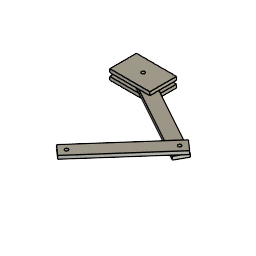
2-Link Manipulator (Autodesk Fusion 360 design; units mm, degrees)
part number: 2025-09-27-21-11-09-060
part number: 2025-09-28-14-52-39-258
part number: 2025-09-28-14-52-39-267
part number: 2025-09-28-14-52-39-272
Autodesk Fusion 360 part; units mm, degrees
sketch "草图1" plane through (0, 0, 0) normal (0, 0, 1) x (1, 0, 0)
  line L0 (30, 20) -> (-30, 20)
  line L1 (-30, 20) -> (-30, -20)
  line L2 (-30, -20) -> (30, -20)
  line L3 (30, -20) -> (30, 20)
  line L4 (30, 20) -> (-30, -20) construction
  line L5 (-30, 20) -> (30, -20) construction
  circle A0 centre (0, 0) radius 2.5
  dimension "d1" = 5
  constraint horizontal L0
  constraint perpendicular L0 L1
  constraint parallel L0 L2
  constraint parallel L1 L3
  constraint coincident L4 A0.centre
  constraint coincident L5 A0.centre
  constraint coincident A0.centre origin
  measures "d1" diameter of A0
sketch "草图3" plane through (0, 0, 0) normal (0, 0, 1) x (1, 0, 0)
  line L0 (59.3105, 8.9123) -> (219.3105, 8.9123)
  line L1 (219.3105, 8.9123) -> (219.3105, -11.0877)
  line L2 (219.3105, -11.0877) -> (59.3105, -11.0877)
  line L3 (59.3105, -11.0877) -> (59.3105, 8.9123)
  circle A0 centre (70, 0) radius 2.5
  circle A1 centre (209.3105, 0) radius 2.5
  dimension "d6" = 160
  dimension "d7" = 20
  dimension "d8" = 5
  dimension "d10" = 5
  constraint horizontal L0
  constraint vertical L1
  constraint horizontal L2
  constraint vertical L3
  measures "d6" distance of L0.start L0.end
  measures "d7" distance of L0.start L2.end
  measures "d8" diameter of A0
  measures "d10" diameter of A1
extrude "拉伸3" add sketch "草图3" along normal blind 5 makes body 1
sketch "草图4" plane through (0, 0, 0) normal (0, 0, 1) x (1, 0, 0)
  line L0 (-33, -75) -> (107, -75)
  line L1 (107, -75) -> (107, -95)
  line L2 (107, -95) -> (-33, -95)
  line L3 (-33, -95) -> (-33, -75)
  circle A0 centre (-23, -85) radius 2.5
  circle A1 centre (97, -85) radius 2.5
  dimension "d13" = 140
  dimension "d14" = 20
  dimension "d15" = 5
  dimension "d16" = 5
  constraint horizontal L0
  constraint vertical L1
  constraint horizontal L2
  constraint vertical L3
  measures "d13" distance of L0.start L0.end
  measures "d14" distance of L0.start L2.end
  measures "d15" diameter of A0
  measures "d16" diameter of A1
extrude "拉伸4" add sketch "草图4" along normal blind 5 separate body makes body 2
sketch "草图5" plane through (0, 0, 0) normal (0, 0, 1) x (1, 0, 0)
  line L0 (-30, 20) -> (30, 20)
  line L1 (30, 20) -> (30, -20)
  line L2 (30, -20) -> (-30, -20)
  line L3 (-30, -20) -> (-30, 20)
  line L4 (-30, 20) -> (30, -20) construction
  line L5 (30, 20) -> (-30, -20) construction
  circle A0 centre (0, 0) radius 2.5
  dimension "d19" = 60
  dimension "d20" = 40
  dimension "d21" = 5
  constraint horizontal L0
  constraint perpendicular L0 L1
  constraint parallel L0 L2
  constraint parallel L1 L3
  constraint coincident L4 A0.centre
  constraint coincident L5 A0.centre
  constraint coincident A0.centre origin
  measures "d19" distance of L1.end L2.end
  measures "d20" distance of L0.end L1.end
  measures "d21" diameter of A0
extrude "拉伸5" add sketch "草图5" along normal blind 5 separate body makes body 3
sketch "草图6" plane through (0, 0, 0) normal (0, 0, 1) x (1, 0, 0)
  circle A0 centre (76.9556, 57.3858) radius 2.5
  dimension "d24" = 5
  measures "d24" diameter of A0
copy_body "实体->零部件1" bodies 3 removing the originals makes body 4 in component "Base"
copy_body "实体->零部件2" bodies 1 removing the originals makes body 5 in component "Link 1"
copy_body "实体->零部件3" bodies 2 removing the originals makes body 6 in component "Link 2"
component "Base" placed x (1, 0, 0) y (0, 1, 0) z (0, 0, 1) at (15.5805, 5.8238, 2.9887)
component "Link 1" placed x (0.721751, -0.692152, 0) y (0.692152, 0.721751, 0) z (0, 0, 1) at (-34.9421, 54.2745, 7.9887)
component "Link 2" placed x (-0.477229, -0.878779, 0) y (0.878779, -0.477229, 0) z (0, 0, 1) at (179.848, -151.3766, 12.9887)
component "Base" placed x (1, 0, 0) y (0, 1, 0) z (0, 0, 1) at (15.5805, 5.8238, 12.9887)
named bodies: "Link 1", "Link 2", "Base"
